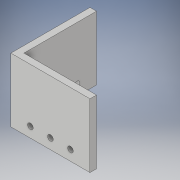
# Autodesk Inventor part: xIdler
Saved by Autodesk Inventor 2019 (Build 230136000, 136)
## iProperties
Created: 2019-05-16
Part Number: xIdler
Material: Generic
Document SubType Name: Modeling
Designer: Alex Jones
Density: 1 g/cm^3
Appearance: Default
Author: Alex Jones
Autodesk Inventor part; units mm, degrees
ref_plane "YZ Plane" through (0, 0, 0) normal (1, 0, 0) x (0, 1, 0)
ref_plane "XZ Plane" through (0, 0, 0) normal (0, 1, 0) x (-1, 0, 0)
ref_plane "XY Plane" through (0, 0, 0) normal (0, 0, 1) x (1, 0, 0)
sketch "Sketch1" plane through (0, 0, 0) normal (0, 1, 0) x (-1, 0, 0)
  line L0 (-25.4, -25.4) -> (25.4, -25.4) construction
  line L1 (25.4, -25.4) -> (25.4, 25.4) construction
  line L2 (25.4, 25.4) -> (-25.4, 25.4) construction
  line L3 (-25.4, 25.4) -> (-25.4, -25.4) construction
  line L4 (-25.4, -25.4) -> (25.4, 25.4) construction
  line L5 (25.4, -25.4) -> (-25.4, 25.4) construction
  line L6 (-25.4, 25.4) -> (25.4, 25.4) construction
  line L7 (25.4, 25.4) -> (25.4, 45.4) construction
  line L8 (25.4, 45.4) -> (-25.4, 45.4)
  line L9 (-25.4, 45.4) -> (-25.4, 25.4) construction
  line L10 (25.4, 45.4) -> (45.4, 45.4)
  line L11 (45.4, 45.4) -> (45.4, -25.4)
  line L12 (45.4, -25.4) -> (25.4, -25.4) construction
  line L13 (25.4, -25.4) -> (25.4, 25.4) construction
  line L14 (25.4, 25.4) -> (25.4, 45.4) construction
  line L15 (-25.4, 45.4) -> (45.4, 45.4)
  line L16 (51.75, 45.4) -> (51.75, 51.75)
  line L17 (51.75, 51.75) -> (-25.4, 51.75)
  line L18 (-25.4, 51.75) -> (-25.4, 45.4)
  line L19 (51.75, 45.4) -> (45.4, 45.4) construction
  line L20 (45.4, 45.4) -> (45.4, -25.4)
  line L21 (45.4, -25.4) -> (51.75, -25.4)
  line L22 (51.75, -25.4) -> (51.75, 45.4)
  line L23 (45.4, 45.4) -> (51.75, 45.4) construction
  point P0 (0, 0)
  dimension "d0" = 50.8
  dimension "d1" = 20
  dimension "d2" = 20
  dimension "d3" = 6.35
  dimension "d4" = 6.35
  constraints: 48 end point, 12 parallel, 7 perpendicular, 6 horizontal, 2 midpoint
  measures "d0" distance of L0.end L1.end
  measures "d1" distance of L11.end L12.end
  measures "d2" distance of L8.end L2.end
  measures "d3" distance of L11.end L21.end
  measures "d4" distance of L17.end L8.end
extrude "Extrusion1" add sketch "Sketch1" along normal blind 62.3
sketch "Sketch2" plane through (-51.75, 0, 51.75) normal (0, 0, 1) x (1, 0, 0)
  line L0 (6.35, 0) -> (0, 0) projected
  line L1 (77.15, 0) -> (77.15, 62.3) projected
  line L2 (0, 0) -> (77.15, 0)
  line L3 (77.15, 0) -> (77.15, 20)
  line L4 (77.15, 20) -> (0, 20)
  line L5 (0, 20) -> (0, 0)
  line L6 (0, 0) -> (0, 62.3) projected
  line L7 (0, 10) -> (77.15, 10) construction
  circle A0 centre (19.05, 10) radius 2.75
  circle A1 centre (38.575, 10) radius 2.75
  circle A2 centre (58.1, 10) radius 2.75
  point P0 (51.75, 0)
  dimension "d7" = 20
  dimension "d8" = 5.5
  dimension "d9" = 19.05
  dimension "d12" = 19.525
  constraints: 10 end point, 3 centre point, 3 point on line, 2 horizontal, 2 parallel, 1 midpoint, 1 perpendicular, 4 other
  measures "d7" distance between parallel lines of L2 L4
  measures "d8" diameter of A0
  measures "d9" distance from line of L5 A0.centre
  measures "d12" distance of A0.centre A1.centre
extrude "Extrusion2" cut sketch "Sketch2" against normal blind 62.3 contours A0 | A1 | A2
sketch "Sketch3" plane through (-51.75, 0, -25.4) normal (-1, 0, 0) x (0, 0, 1)
  circle A0 centre (19.05, 10) radius 2.75
  line L0 (0, 0) -> (77.15, 0) projected
  line L1 (0, 0) -> (0, 62.3) projected
  circle A1 centre (38.575, 10) radius 2.75
  circle A2 centre (58.1, 10) radius 2.75
  point P0 (25.4, 0)
  dimension "d19" = 10
  dimension "d20" = 5.5
  dimension "d21" = 19.05
  dimension "d24" = 19.525
  constraints: 3 centre point, 1 horizontal, 4 other
  measures "d19" distance from line of L0 A0.centre
  measures "d20" diameter of A0
  measures "d21" distance from line of L1 A0.centre
  measures "d24" distance of A0.centre A1.centre
extrude "Extrusion3" cut sketch "Sketch3" against normal blind 62.3
body "Solid1"
